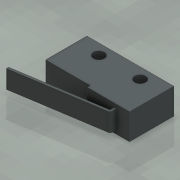
# Autodesk Inventor part: Limit Switch
Saved by Autodesk Inventor 2015 (Build 190159000, 159)
## iProperties
Created: 2015-06-04
Part Number: Limit Switch
Material: Generic
Document SubType Name: Modeling
Designer: pltwe4
Density: 1 g/cm^3
Appearance: Default
Author: pltwe4
Autodesk Inventor part; units mm, degrees
ref_plane "YZ Plane" through (0, 0, 0) normal (1, 0, 0) x (0, 1, 0)
ref_plane "XZ Plane" through (0, 0, 0) normal (0, 1, 0) x (-1, 0, 0)
ref_plane "XY Plane" through (0, 0, 0) normal (0, 0, 1) x (1, 0, 0)
sketch "Sketch1" plane through (0, 0, 0) normal (0, 0, 1) x (1, 0, 0)
  line L0 (10, 4.75) -> (-10, 4.75)
  line L1 (-10, 4.75) -> (-10, -4.75)
  line L2 (-10, -4.75) -> (10, -4.75)
  line L3 (10, -4.75) -> (10, 4.75)
  line L4 (0.25, -4.75) -> (0.25, -5.45)
  line L5 (0.25, -5.45) -> (10, -5.45)
  line L6 (10, -5.45) -> (10, -4.75)
  line L7 (-10, -4.75) -> (10, 4.75) construction
  line L8 (10, -4.75) -> (-10, 4.75) construction
  circle A0 centre (-4.75, 2.25) radius 1.27
  circle A1 centre (4.75, 2.25) radius 1.27
  line L9 (0, 0) -> (0, 4.75) construction
  dimension "d0" = 20
  dimension "d2" = 10.2
  dimension "d3" = 9.5
  dimension "d4" = 9.75
  dimension "d5" = 9.5
  dimension "d6" = 2.54
  dimension "d7" = 2.5
  constraints: 20 end point, 3 midpoint, 3 perpendicular, 2 centre point, 2 parallel, 1 horizontal, 1 point on line, 1 vertical, 1 other
  measures "d0" distance of L0.start L0.end
  measures "d2" distance between parallel lines of L0 L5
  measures "d3" distance between parallel lines of L0 L2
  measures "d4" distance of L4.end L5.end
  measures "d5" distance of A1.centre A0.centre
  measures "d6" diameter of A0
  measures "d7" distance from line of A0.centre L0
extrude "Extrusion1" add sketch "Sketch1" along normal mid plane 6
sketch "Sketch2" plane through (0.25, -5.45, -3) normal (0, -1, 0) x (1, 0, 0)
  line L0 (6.75, 0.9) -> (6.25, 0.9)
  line L1 (6.25, 0.9) -> (6.25, 5.1)
  line L2 (6.25, 5.1) -> (6.75, 5.1)
  line L3 (6.75, 5.1) -> (6.75, 0.9)
  line L4 (-14.25, 3) -> (13.75, 3) projected
  line L5 (9.75, 0) -> (9.75, 6) projected
  point P0 (-0.25, 3)
  dimension "d10" = 4.2
  dimension "d11" = 0.5
  dimension "d12" = 3
  constraints: 8 end point, 2 parallel, 1 horizontal, 1 perpendicular, 1 other
  measures "d10" distance of L2.end L0.start
  measures "d11" distance of L0.start L0.end
  measures "d12" distance between parallel lines of L5 L3
extrude "Extrusion2" add sketch "Sketch2" along normal blind 1
sketch "Sketch3" plane through (6.5, -5.45, 2.1) normal (0, 0, 1) x (1, 0, 0)
  line L0 (0, -1) -> (-20.256, -4.1472)
  line L1 (-20.256, -4.1472) -> (-20.1793, -4.6413)
  line L2 (-20.1793, -4.6413) -> (0.0768, -1.4941)
  arc A0 (0.0768, -1.4941) -> (0.5, -1) centre (0, -1) ccw
  line L3 (0.5, -1) -> (0, -1) projected
  point P0 (-6.5, 5.45)
  dimension "d15" = 0.5
  constraints: 6 end point, 2 perpendicular, 2 point on circle, 1 centre point, 1 coincident, 1 point on line, 1 tangent
  measures "d15" distance between parallel lines of L0 L2
extrude "Extrusion3" add sketch "Sketch3" against normal blind 4.2
body "Solid1"
